Autodesk Fusion 360 part; units mm, degrees
note: some values were not read from the file. Chosen so that the rebuilt part matches the saved one: which bodies a step acts on.
(part 5 of 5)
sketch "スケッチ4 (17)" plane through (0, 0, 0) normal (0, 0, 1) x (1, 0, 0) in component "Stage2_Internal_Ring_Gear"
  circle A0 centre (62, 0) radius 3
  circle A1 centre (43.8406, 43.8406) radius 3
  circle A2 centre (0, 62) radius 3
  circle A3 centre (-43.8406, 43.8406) radius 3
  circle A4 centre (-62, 0) radius 3
  circle A5 centre (-43.8406, -43.8406) radius 3
  circle A6 centre (0, -62) radius 3
  circle A7 centre (43.8406, -43.8406) radius 3
extrude "Stage2_Ring_Bolt_Hole_Cut" cut sketch "スケッチ4 (17)" along normal blind 8 from surface at 76 bodies 19 in component "Stage2_Internal_Ring_Gear"
sketch "スケッチ5 (8)" plane through (0, 0, 0) normal (0, 0, 1) x (1, 0, 0) in component "Stage2_Internal_Ring_Gear"
  circle A0 centre (51.1941, 13.7174) radius 3.5
  circle A1 centre (37.4767, 37.4767) radius 3.5
  circle A2 centre (13.7174, 51.1941) radius 3.5
  circle A3 centre (-13.7174, 51.1941) radius 3.5
  circle A4 centre (-37.4767, 37.4767) radius 3.5
  circle A5 centre (-51.1941, 13.7174) radius 3.5
  circle A6 centre (-51.1941, -13.7174) radius 3.5
  circle A7 centre (-37.4767, -37.4767) radius 3.5
  circle A8 centre (-13.7174, -51.1941) radius 3.5
  circle A9 centre (13.7174, -51.1941) radius 3.5
  circle A10 centre (37.4767, -37.4767) radius 3.5
  circle A11 centre (51.1941, -13.7174) radius 3.5
extrude "Stage2_Ring_Lightening_Cut" cut sketch "スケッチ5 (8)" along normal blind 15 from surface at 73 bodies 19 in component "Stage2_Internal_Ring_Gear"
sketch "スケッチ1 (19)" plane through (0, 0, 0) normal (0, 0, 1) x (1, 0, 0) in component "Stage2_Output_Carrier"
  circle A0 centre (0, 0) radius 38
extrude "Stage2_Carrier_Lower_Plate_Extrude" add sketch "スケッチ1 (19)" along normal blind 5 from surface at 66 separate body makes body 20 in component "Stage2_Output_Carrier"
sketch "スケッチ2 (19)" plane through (0, 0, 0) normal (0, 0, 1) x (1, 0, 0) in component "Stage2_Output_Carrier"
  circle A0 centre (0, 0) radius 16
extrude "Stage2_Carrier_Lower_Bore_Cut" cut sketch "スケッチ2 (19)" along normal blind 7 from surface at 65 bodies 20 in component "Stage2_Output_Carrier"
sketch "スケッチ3 (18)" plane through (0, 0, 0) normal (0, 0, 1) x (1, 0, 0) in component "Stage2_Output_Carrier"
  circle A0 centre (21.2132, 21.2132) radius 5.5
  circle A1 centre (-21.2132, 21.2132) radius 5.5
  circle A2 centre (-21.2132, -21.2132) radius 5.5
  circle A3 centre (21.2132, -21.2132) radius 5.5
extrude "Stage2_Carrier_Post_Extrude" add sketch "スケッチ3 (18)" along normal blind 19 from surface at 71 bodies 20 in component "Stage2_Output_Carrier"
sketch "スケッチ4 (18)" plane through (0, 0, 0) normal (0, 0, 1) x (1, 0, 0) in component "Stage2_Output_Carrier"
  circle A0 centre (0, 0) radius 38
extrude "Stage2_Carrier_Output_Plate_Extrude" add sketch "スケッチ4 (18)" along normal blind 7 from surface at 90 bodies 20 in component "Stage2_Output_Carrier"
sketch "スケッチ5 (9)" plane through (0, 0, 0) normal (0, 0, 1) x (1, 0, 0) in component "Stage2_Output_Carrier"
  circle A0 centre (0, 0) radius 18
extrude "Stage2_Carrier_Hub_Extrude" add sketch "スケッチ5 (9)" along normal blind 6 from surface at 97 bodies 20 in component "Stage2_Output_Carrier"
sketch "スケッチ6 (4)" plane through (0, 0, 0) normal (0, 0, 1) x (1, 0, 0) in component "Stage2_Output_Carrier"
  circle A0 centre (35.1074, 14.542) radius 6
  circle A1 centre (14.542, 35.1074) radius 6
  circle A2 centre (-14.542, 35.1074) radius 6
  circle A3 centre (-35.1074, 14.542) radius 6
  circle A4 centre (-35.1074, -14.542) radius 6
  circle A5 centre (-14.542, -35.1074) radius 6
  circle A6 centre (14.542, -35.1074) radius 6
  circle A7 centre (35.1074, -14.542) radius 6
extrude "Stage2_Carrier_Lightening_Cut" cut sketch "スケッチ6 (4)" along normal blind 33 from surface at 65 bodies 20 in component "Stage2_Output_Carrier"
sketch "スケッチ7 (3)" plane through (0, 0, 0) normal (0, 0, 1) x (1, 0, 0) in component "Stage2_Output_Carrier"
  circle A0 centre (30, 0) radius 4.1
  circle A1 centre (0, 30) radius 4.1
  circle A2 centre (-30, 0) radius 4.1
  circle A3 centre (0, -30) radius 4.1
extrude "Stage2_Carrier_Pin_Hole_Cut" cut sketch "スケッチ7 (3)" along normal blind 33 from surface at 65 bodies 20 in component "Stage2_Output_Carrier"
sketch "スケッチ1 (20)" plane through (0, 0, 0) normal (0, 0, 1) x (1, 0, 0) in component "Output_Shaft"
  circle A0 centre (0, 0) radius 12
extrude "Output_Shaft_Main_Extrude" add sketch "スケッチ1 (20)" along normal blind 35 from surface at 99 separate body makes body 21 in component "Output_Shaft"
sketch "スケッチ2 (20)" plane through (0, 0, 0) normal (0, 0, 1) x (1, 0, 0) in component "Output_Shaft"
  circle A0 centre (0, 0) radius 15
extrude "Output_Shaft_Bearing_Seat_Extrude" add sketch "スケッチ2 (20)" along normal blind 10 from surface at 106 bodies 21 in component "Output_Shaft"
sketch "スケッチ3 (19)" plane through (0, 0, 0) normal (0, 0, 1) x (1, 0, 0) in component "Output_Shaft"
  line L0 (-3, 10) -> (3, 10)
  line L1 (3, 10) -> (3, 12.5)
  line L2 (3, 12.5) -> (-3, 12.5)
  line L3 (-3, 12.5) -> (-3, 10)
extrude "Output_Shaft_Keyway_Cut" cut sketch "スケッチ3 (19)" along normal blind 15 from surface at 119 bodies 21 in component "Output_Shaft"
sketch "スケッチ1 (21)" plane through (0, 0, 0) normal (0, 0, 1) x (1, 0, 0) in component "Output_Flange"
  circle A0 centre (0, 0) radius 18
extrude "Output_Flange_Hub_Extrude" add sketch "スケッチ1 (21)" along normal blind 6 from surface at 128 separate body makes body 22 in component "Output_Flange"
sketch "スケッチ2 (21)" plane through (0, 0, 0) normal (0, 0, 1) x (1, 0, 0) in component "Output_Flange"
  circle A0 centre (0, 0) radius 40
extrude "Output_Flange_Plate_Extrude" add sketch "スケッチ2 (21)" along normal blind 8 from surface at 134 bodies 22 in component "Output_Flange"
sketch "スケッチ3 (20)" plane through (0, 0, 0) normal (0, 0, 1) x (1, 0, 0) in component "Output_Flange"
  circle A0 centre (0, 0) radius 12.15
extrude "Output_Flange_Bore_Cut" cut sketch "スケッチ3 (20)" along normal blind 10 from surface at 127 bodies 22 in component "Output_Flange"
sketch "スケッチ4 (19)" plane through (0, 0, 0) normal (0, 0, 1) x (1, 0, 0) in component "Output_Flange"
  circle A0 centre (32, 0) radius 4
  circle A1 centre (22.6274, 22.6274) radius 4
  circle A2 centre (0, 32) radius 4
  circle A3 centre (-22.6274, 22.6274) radius 4
  circle A4 centre (-32, 0) radius 4
  circle A5 centre (-22.6274, -22.6274) radius 4
  circle A6 centre (0, -32) radius 4
  circle A7 centre (22.6274, -22.6274) radius 4
extrude "Output_Flange_Bolt_Hole_Cut" cut sketch "スケッチ4 (19)" along normal blind 10 from surface at 133 bodies 22 in component "Output_Flange"
sketch "スケッチ5 (10)" plane through (0, 0, 0) normal (0, 0, 1) x (1, 0, 0) in component "Output_Flange"
  circle A0 centre (21.2504, 5.694) radius 2.5
  circle A1 centre (15.5563, 15.5563) radius 2.5
  circle A2 centre (5.694, 21.2504) radius 2.5
  circle A3 centre (-5.694, 21.2504) radius 2.5
  circle A4 centre (-15.5563, 15.5563) radius 2.5
  circle A5 centre (-21.2504, 5.694) radius 2.5
  circle A6 centre (-21.2504, -5.694) radius 2.5
  circle A7 centre (-15.5563, -15.5563) radius 2.5
  circle A8 centre (-5.694, -21.2504) radius 2.5
  circle A9 centre (5.694, -21.2504) radius 2.5
  circle A10 centre (15.5563, -15.5563) radius 2.5
  circle A11 centre (21.2504, -5.694) radius 2.5
extrude "Output_Flange_Index_Hole_Cut" cut sketch "スケッチ5 (10)" along normal blind 10 from surface at 133 bodies 22 in component "Output_Flange"
sketch "スケッチ8" plane through (0, 0, 0) normal (0, 0, 1) x (1, 0, 0) in component "Lower_Base_Plate"
  circle A0 centre (0, 0) radius 22.3
extrude "Base_Bearing_Counterbore_Cut" cut sketch "スケッチ8" along normal blind 7 from surface at 13 bodies 1 in component "Lower_Base_Plate"
sketch "スケッチ8 (2)" plane through (0, 0, 0) normal (0, 0, 1) x (1, 0, 0) in component "Stage1_Planet_Carrier"
  circle A0 centre (0, 0) radius 23
extrude "Stage1_Carrier_Bore_Relief_Cut" cut sketch "スケッチ8 (2)" along normal blind 8 from surface at 23 bodies 11 in component "Stage1_Planet_Carrier"
sketch "スケッチ1 (22)" plane through (0, 0, 0) normal (0, 0, 1) x (1, 0, 0) in component "Bearing_Set"
  circle A0 centre (0, 0) radius 22
extrude "Input_Bearing_Outer_Race_Extrude" add sketch "スケッチ1 (22)" along normal blind 10 from surface at 15 separate body makes body 23 in component "Bearing_Set"
sketch "スケッチ2 (22)" plane through (0, 0, 0) normal (0, 0, 1) x (1, 0, 0) in component "Bearing_Set"
  circle A0 centre (0, 0) radius 20.6
extrude "Input_Bearing_Outer_Race_Bore_Cut" cut sketch "スケッチ2 (22)" along normal blind 12 from surface at 14 bodies 23 in component "Bearing_Set"
sketch "スケッチ3 (21)" plane through (0, 0, 0) normal (0, 0, 1) x (1, 0, 0) in component "Bearing_Set"
  circle A0 centre (0, 0) radius 20.4
extrude "Input_Bearing_Cage_Extrude" add sketch "スケッチ3 (21)" along normal blind 6 from surface at 17 separate body makes body 24 in component "Bearing_Set"
sketch "スケッチ4 (20)" plane through (0, 0, 0) normal (0, 0, 1) x (1, 0, 0) in component "Bearing_Set"
  circle A0 centre (0, 0) radius 18.6
extrude "Input_Bearing_Cage_Bore_Cut" cut sketch "スケッチ4 (20)" along normal blind 8 from surface at 16 bodies 24 in component "Bearing_Set"
sketch "スケッチ5 (11)" plane through (0, 0, 0) normal (0, 0, 1) x (1, 0, 0) in component "Bearing_Set"
  circle A0 centre (0, 0) radius 18.4
extrude "Input_Bearing_Inner_Race_Extrude" add sketch "スケッチ5 (11)" along normal blind 10 from surface at 15 separate body makes body 25 in component "Bearing_Set"
sketch "スケッチ6 (5)" plane through (0, 0, 0) normal (0, 0, 1) x (1, 0, 0) in component "Bearing_Set"
  circle A0 centre (0, 0) radius 13.1
extrude "Input_Bearing_Inner_Race_Bore_Cut" cut sketch "スケッチ6 (5)" along normal blind 12 from surface at 14 bodies 25 in component "Bearing_Set"
sketch "スケッチ7 (4)" plane through (0, 0, 0) normal (0, 0, 1) x (1, 0, 0) in component "Bearing_Set"
  circle A0 centre (0, 0) radius 23.8
extrude "Intermediate_Bearing_Outer_Race_Extrude" add sketch "スケッチ7 (4)" along normal blind 6 from surface at 57 separate body makes body 26 in component "Bearing_Set"
sketch "スケッチ8 (3)" plane through (0, 0, 0) normal (0, 0, 1) x (1, 0, 0) in component "Bearing_Set"
  circle A0 centre (0, 0) radius 22.4
extrude "Intermediate_Bearing_Outer_Race_Bore_Cut" cut sketch "スケッチ8 (3)" along normal blind 8 from surface at 56 bodies 26 in component "Bearing_Set"
sketch "スケッチ9" plane through (0, 0, 0) normal (0, 0, 1) x (1, 0, 0) in component "Bearing_Set"
  circle A0 centre (0, 0) radius 22.2
extrude "Intermediate_Bearing_Cage_Extrude" add sketch "スケッチ9" along normal blind 4 from surface at 58 separate body makes body 27 in component "Bearing_Set"
sketch "スケッチ10" plane through (0, 0, 0) normal (0, 0, 1) x (1, 0, 0) in component "Bearing_Set"
  circle A0 centre (0, 0) radius 20.4
extrude "Intermediate_Bearing_Cage_Bore_Cut" cut sketch "スケッチ10" along normal blind 6 from surface at 57 bodies 27 in component "Bearing_Set"
sketch "スケッチ11" plane through (0, 0, 0) normal (0, 0, 1) x (1, 0, 0) in component "Bearing_Set"
  circle A0 centre (0, 0) radius 20.2
extrude "Intermediate_Bearing_Inner_Race_Extrude" add sketch "スケッチ11" along normal blind 6 from surface at 57 separate body makes body 28 in component "Bearing_Set"
sketch "スケッチ12" plane through (0, 0, 0) normal (0, 0, 1) x (1, 0, 0) in component "Bearing_Set"
  circle A0 centre (0, 0) radius 16.2
extrude "Intermediate_Bearing_Inner_Race_Bore_Cut" cut sketch "スケッチ12" along normal blind 8 from surface at 56 bodies 28 in component "Bearing_Set"
sketch "スケッチ13" plane through (0, 0, 0) normal (0, 0, 1) x (1, 0, 0) in component "Bearing_Set"
  circle A0 centre (0, 0) radius 23.5
extrude "Output_Bearing_Outer_Race_Extrude" add sketch "スケッチ13" along normal blind 10 from surface at 106 separate body makes body 29 in component "Bearing_Set"
sketch "スケッチ14" plane through (0, 0, 0) normal (0, 0, 1) x (1, 0, 0) in component "Bearing_Set"
  circle A0 centre (0, 0) radius 22.1
extrude "Output_Bearing_Outer_Race_Bore_Cut" cut sketch "スケッチ14" along normal blind 12 from surface at 105 bodies 29 in component "Bearing_Set"
sketch "スケッチ15" plane through (0, 0, 0) normal (0, 0, 1) x (1, 0, 0) in component "Bearing_Set"
  circle A0 centre (0, 0) radius 21.9
extrude "Output_Bearing_Cage_Extrude" add sketch "スケッチ15" along normal blind 6 from surface at 108 separate body makes body 30 in component "Bearing_Set"
sketch "スケッチ16" plane through (0, 0, 0) normal (0, 0, 1) x (1, 0, 0) in component "Bearing_Set"
  circle A0 centre (0, 0) radius 20.1
extrude "Output_Bearing_Cage_Bore_Cut" cut sketch "スケッチ16" along normal blind 8 from surface at 107 bodies 30 in component "Bearing_Set"
sketch "スケッチ17" plane through (0, 0, 0) normal (0, 0, 1) x (1, 0, 0) in component "Bearing_Set"
  circle A0 centre (0, 0) radius 19.9
extrude "Output_Bearing_Inner_Race_Extrude" add sketch "スケッチ17" along normal blind 10 from surface at 106 separate body makes body 31 in component "Bearing_Set"
sketch "スケッチ18" plane through (0, 0, 0) normal (0, 0, 1) x (1, 0, 0) in component "Bearing_Set"
  circle A0 centre (0, 0) radius 15.1
extrude "Output_Bearing_Inner_Race_Bore_Cut" cut sketch "スケッチ18" along normal blind 12 from surface at 105 bodies 31 in component "Bearing_Set"
sketch "スケッチ1 (23)" plane through (0, 0, 0) normal (0, 0, 1) x (1, 0, 0) in component "Planet_Pin_Set"
  circle A0 centre (31.5, 0) radius 4
  circle A1 centre (-15.75, 27.2798) radius 4
  circle A2 centre (-15.75, -27.2798) radius 4
extrude "Stage1_Planet_Pin_Extrude" add sketch "スケッチ1 (23)" along normal blind 35.8 from surface at 22 separate body makes body 32 at (35.4801, -0.3983, 33.9333) makes body 33 at (-11.7699, 26.8815, 33.9333) makes body 34 at (-11.7699, -27.6781, 33.9333) in component "Planet_Pin_Set"
sketch "スケッチ2 (23)" plane through (0, 0, 0) normal (0, 0, 1) x (1, 0, 0) in component "Planet_Pin_Set"
  circle A0 centre (31.5, 0) radius 8
  circle A1 centre (-15.75, 27.2798) radius 8
  circle A2 centre (-15.75, -27.2798) radius 8
extrude "Stage1_Pin_Washer_Lower_Extrude" add sketch "スケッチ2 (23)" along normal blind 2 from surface at 20 bodies 32 33 34 in component "Planet_Pin_Set"
sketch "スケッチ3 (22)" plane through (0, 0, 0) normal (0, 0, 1) x (1, 0, 0) in component "Planet_Pin_Set"
  circle A0 centre (31.5, 0) radius 6.5
  circle A1 centre (-15.75, 27.2798) radius 6.5
  circle A2 centre (-15.75, -27.2798) radius 6.5
extrude "Stage1_Pin_Collar_Upper_Extrude" add sketch "スケッチ3 (22)" along normal blind 1.8 from surface at 56 bodies 32 33 34 in component "Planet_Pin_Set"
sketch "スケッチ4 (21)" plane through (0, 0, 0) normal (0, 0, 1) x (1, 0, 0) in component "Planet_Pin_Set"
  circle A0 centre (30, 0) radius 4
  circle A1 centre (0, 30) radius 4
  circle A2 centre (-30, 0) radius 4
  circle A3 centre (0, -30) radius 4
extrude "Stage2_Planet_Pin_Extrude" add sketch "スケッチ4 (21)" along normal blind 33 from surface at 64 separate body makes body 35 at (-26.0199, -0.3983, 86) makes body 36 at (3.9801, 29.6017, 86) makes body 37 at (33.9801, -0.3983, 86) makes body 38 at (3.9801, -30.3983, 86) in component "Planet_Pin_Set"
sketch "スケッチ5 (12)" plane through (0, 0, 0) normal (0, 0, 1) x (1, 0, 0) in component "Planet_Pin_Set"
  circle A0 centre (30, 0) radius 8
  circle A1 centre (0, 30) radius 8
  circle A2 centre (-30, 0) radius 8
  circle A3 centre (0, -30) radius 8
extrude "Stage2_Pin_Washer_Lower_Extrude" add sketch "スケッチ5 (12)" along normal blind 2 from surface at 62 bodies 32 33 34 35 36 37 38 in component "Planet_Pin_Set"
sketch "スケッチ6 (6)" plane through (0, 0, 0) normal (0, 0, 1) x (1, 0, 0) in component "Planet_Pin_Set"
  line L0 (36.6, 0) -> (33.3, 5.7158)
  line L1 (33.3, 5.7158) -> (26.7, 5.7158)
  line L2 (26.7, 5.7158) -> (23.4, 0)
  line L3 (23.4, 0) -> (26.7, -5.7158)
  line L4 (26.7, -5.7158) -> (33.3, -5.7158)
  line L5 (33.3, -5.7158) -> (36.6, 0)
  line L6 (6.6, 30) -> (3.3, 35.7158)
  line L7 (3.3, 35.7158) -> (-3.3, 35.7158)
  line L8 (-3.3, 35.7158) -> (-6.6, 30)
  line L9 (-6.6, 30) -> (-3.3, 24.2842)
  line L10 (-3.3, 24.2842) -> (3.3, 24.2842)
  line L11 (3.3, 24.2842) -> (6.6, 30)
  line L12 (-23.4, 0) -> (-26.7, 5.7158)
  line L13 (-26.7, 5.7158) -> (-33.3, 5.7158)
  line L14 (-33.3, 5.7158) -> (-36.6, 0)
  line L15 (-36.6, 0) -> (-33.3, -5.7158)
  line L16 (-33.3, -5.7158) -> (-26.7, -5.7158)
  line L17 (-26.7, -5.7158) -> (-23.4, 0)
  line L18 (6.6, -30) -> (3.3, -24.2842)
  line L19 (3.3, -24.2842) -> (-3.3, -24.2842)
  line L20 (-3.3, -24.2842) -> (-6.6, -30)
  line L21 (-6.6, -30) -> (-3.3, -35.7158)
  line L22 (-3.3, -35.7158) -> (3.3, -35.7158)
  line L23 (3.3, -35.7158) -> (6.6, -30)
extrude "Stage2_Pin_Nut_Extrude" add sketch "スケッチ6 (6)" along normal blind 5 from surface at 97 bodies 32 33 34 35 36 37 38 in component "Planet_Pin_Set"
sketch "スケッチ1 (24)" plane through (0, 0, 0) normal (0, 0, 1) x (1, 0, 0) in component "Housing_Tie_Rods"
  circle A0 centre (75, 0) radius 4
extrude "Housing_TieRod_Extrude" add sketch "スケッチ1 (24)" along normal blind 101 from surface at 14 separate body makes body 39 in component "Housing_Tie_Rods"
pattern_circular "Housing_TieRod_Pattern" count 8 over 360 about axis through (0, 0, 1.75) along (0, 0, 1) of bodies 39 makes body 40 at (55.9989, 55.7169, 81.3333) makes body 41 at (0.1994, 78.995, 81.3333) makes body 42 at (-55.7169, 55.9989, 81.3333) makes body 43 at (-78.995, 0.1994, 81.3333) makes body 44 at (-55.9989, -55.7169, 81.3333) makes body 45 at (-0.1994, -78.995, 81.3333) makes body 46 at (55.7169, -55.9989, 81.3333) in component "Housing_Tie_Rods"
sketch "スケッチ1 (25)" plane through (0, 0, 0) normal (0, 0, 1) x (1, 0, 0) in component "Fastener_Set"
  circle A0 centre (75, 0) radius 9
extrude "TieRod_Lower_Washer_Extrude" add sketch "スケッチ1 (25)" along normal blind 1.6 from surface at 20 separate body makes body 47 in component "Fastener_Set"
sketch "スケッチ2 (24)" plane through (0, 0, 0) normal (0, 0, 1) x (1, 0, 0) in component "Fastener_Set"
  line L0 (83.1, 0) -> (79.05, 7.0148)
  line L1 (79.05, 7.0148) -> (70.95, 7.0148)
  line L2 (70.95, 7.0148) -> (66.9, 0)
  line L3 (66.9, 0) -> (70.95, -7.0148)
  line L4 (70.95, -7.0148) -> (79.05, -7.0148)
  line L5 (79.05, -7.0148) -> (83.1, 0)
extrude "TieRod_Lower_Nut_Extrude" add sketch "スケッチ2 (24)" along normal blind 7 from surface at 21.6 separate body makes body 48 in component "Fastener_Set"
sketch "スケッチ3 (23)" plane through (0, 0, 0) normal (0, 0, 1) x (1, 0, 0) in component "Fastener_Set"
  circle A0 centre (75, 0) radius 9
extrude "TieRod_Upper_Washer_Extrude" add sketch "スケッチ3 (23)" along normal blind 1.6 from surface at 104 separate body makes body 49 in component "Fastener_Set"
sketch "スケッチ4 (22)" plane through (0, 0, 0) normal (0, 0, 1) x (1, 0, 0) in component "Fastener_Set"
  line L0 (83.1, 0) -> (79.05, 7.0148)
  line L1 (79.05, 7.0148) -> (70.95, 7.0148)
  line L2 (70.95, 7.0148) -> (66.9, 0)
  line L3 (66.9, 0) -> (70.95, -7.0148)
  line L4 (70.95, -7.0148) -> (79.05, -7.0148)
  line L5 (79.05, -7.0148) -> (83.1, 0)
extrude "TieRod_Upper_Nut_Extrude" add sketch "スケッチ4 (22)" along normal blind 7 from surface at 105.6 separate body makes body 50 in component "Fastener_Set"
pattern_circular "Fastener_Circular_Pattern" count 8 over 360 about axis through (0, 0, 1.75) along (0, 0, 1) of bodies 47 48 49 50 makes body 51 at (48.1121, 50.7772, 20) makes body 52 at (2.4777, 78.6341, 20) makes body 53 at (-51.2227, 48.0619, 20) makes body 54 at (-78.6341, 2.4777, 20) makes body 55 at (-49.9226, -53.9664, 20) makes body 56 at (-2.4777, -78.6341, 20) makes body 57 at (50.7772, -48.1121, 20) makes body 58 at (52.3342, 55.641, 28.6) makes body 59 at (-2.3383, 76.35, 28.6) makes body 60 at (-53.7318, 50.425, 28.6) makes body 61 at (-76.35, -2.3383, 28.6) makes body 62 at (-52.3342, -55.641, 28.6) makes body 63 at (2.3383, -76.35, 28.6) makes body 64 at (55.641, -52.3342, 28.6) makes body 65 at (48.1121, 50.7772, 104) makes body 66 at (2.4777, 78.6341, 104) makes body 67 at (-51.2227, 48.0619, 104) makes body 68 at (-78.6341, 2.4777, 104) makes body 69 at (-49.9226, -53.9664, 104) makes body 70 at (-2.4777, -78.6341, 104) makes body 71 at (50.7772, -48.1121, 104) makes body 72 at (52.3342, 55.641, 112.6) makes body 73 at (-2.3383, 76.35, 112.6) makes body 74 at (-53.7318, 50.425, 112.6) makes body 75 at (-76.35, -2.3383, 112.6) makes body 76 at (-52.3342, -55.641, 112.6) makes body 77 at (2.3383, -76.35, 112.6) makes body 78 at (55.641, -52.3342, 112.6) in component "Fastener_Set"
sketch "スケッチ1 (26)" plane through (0, 0, 0) normal (0, 0, 1) x (1, 0, 0) in component "Transparent_Outer_Housing"
  circle A0 centre (0, 0) radius 69
extrude "Outer_Housing_Wall_Extrude" add sketch "スケッチ1 (26)" along normal blind 74 from surface at 30 separate body makes body 79 in component "Transparent_Outer_Housing"
sketch "スケッチ2 (25)" plane through (0, 0, 0) normal (0, 0, 1) x (1, 0, 0) in component "Transparent_Outer_Housing"
  circle A0 centre (0, 0) radius 80
extrude "Outer_Housing_Lower_Flange_Extrude" add sketch "スケッチ2 (25)" along normal blind 8 from surface at 30 bodies 79 in component "Transparent_Outer_Housing"
sketch "スケッチ3 (24)" plane through (0, 0, 0) normal (0, 0, 1) x (1, 0, 0) in component "Transparent_Outer_Housing"
  circle A0 centre (0, 0) radius 80
extrude "Outer_Housing_Upper_Flange_Extrude" add sketch "スケッチ3 (24)" along normal blind 8 from surface at 96 bodies 79 in component "Transparent_Outer_Housing"
sketch "スケッチ4 (23)" plane through (0, 0, 0) normal (0, 0, 1) x (1, 0, 0) in component "Transparent_Outer_Housing"
  line L0 (62.3154, 22.0235) -> (68.7826, 24.7023)
  line L1 (68.7826, 24.7023) -> (66.1038, 31.1695)
  line L2 (66.1038, 31.1695) -> (59.6367, 28.4907)
  line L3 (59.6367, 28.4907) -> (62.3154, 22.0235)
  line L4 (28.4907, 59.6367) -> (31.1695, 66.1038)
  line L5 (31.1695, 66.1038) -> (24.7023, 68.7826)
  line L6 (24.7023, 68.7826) -> (22.0235, 62.3154)
  line L7 (22.0235, 62.3154) -> (28.4907, 59.6367)
  line L8 (-22.0235, 62.3154) -> (-24.7023, 68.7826)
  line L9 (-24.7023, 68.7826) -> (-31.1695, 66.1038)
  line L10 (-31.1695, 66.1038) -> (-28.4907, 59.6367)
  line L11 (-28.4907, 59.6367) -> (-22.0235, 62.3154)
  line L12 (-59.6367, 28.4907) -> (-66.1038, 31.1695)
  line L13 (-66.1038, 31.1695) -> (-68.7826, 24.7023)
  line L14 (-68.7826, 24.7023) -> (-62.3154, 22.0235)
  line L15 (-62.3154, 22.0235) -> (-59.6367, 28.4907)
  line L16 (-62.3154, -22.0235) -> (-68.7826, -24.7023)
  line L17 (-68.7826, -24.7023) -> (-66.1038, -31.1695)
  line L18 (-66.1038, -31.1695) -> (-59.6367, -28.4907)
  line L19 (-59.6367, -28.4907) -> (-62.3154, -22.0235)
  line L20 (-28.4907, -59.6367) -> (-31.1695, -66.1038)
  line L21 (-31.1695, -66.1038) -> (-24.7023, -68.7826)
  line L22 (-24.7023, -68.7826) -> (-22.0235, -62.3154)
  line L23 (-22.0235, -62.3154) -> (-28.4907, -59.6367)
  line L24 (22.0235, -62.3154) -> (24.7023, -68.7826)
  line L25 (24.7023, -68.7826) -> (31.1695, -66.1038)
  line L26 (31.1695, -66.1038) -> (28.4907, -59.6367)
  line L27 (28.4907, -59.6367) -> (22.0235, -62.3154)
  line L28 (59.6367, -28.4907) -> (66.1038, -31.1695)
  line L29 (66.1038, -31.1695) -> (68.7826, -24.7023)
  line L30 (68.7826, -24.7023) -> (62.3154, -22.0235)
  line L31 (62.3154, -22.0235) -> (59.6367, -28.4907)
extrude "Outer_Housing_Rib_Extrude" add sketch "スケッチ4 (23)" along normal blind 58 from surface at 38 bodies 79 in component "Transparent_Outer_Housing"
sketch "スケッチ5 (13)" plane through (0, 0, 0) normal (0, 0, 1) x (1, 0, 0) in component "Transparent_Outer_Housing"
  circle A0 centre (0, 0) radius 66
extrude "Outer_Housing_Bore_Cut" cut sketch "スケッチ5 (13)" along normal blind 76 from surface at 29 bodies 79 in component "Transparent_Outer_Housing"
sketch "スケッチ6 (7)" plane through (0, 0, 0) normal (0, 0, 1) x (1, 0, 0) in component "Transparent_Outer_Housing"
  circle A0 centre (75, 0) radius 4.6
  circle A1 centre (53.033, 53.033) radius 4.6
  circle A2 centre (0, 75) radius 4.6
  circle A3 centre (-53.033, 53.033) radius 4.6
  circle A4 centre (-75, 0) radius 4.6
  circle A5 centre (-53.033, -53.033) radius 4.6
  circle A6 centre (0, -75) radius 4.6
  circle A7 centre (53.033, -53.033) radius 4.6
extrude "Outer_Housing_Bolt_Hole_Cut" cut sketch "スケッチ6 (7)" along normal blind 76 from surface at 29 bodies 79 in component "Transparent_Outer_Housing"
fillet "Base_Plate_Edge_Fillet" radius 3 2 edges at (-78.3155, -30.3757, 14) (-78.3155, -30.3757, 0) on bodies 1 in component "Lower_Base_Plate"
fillet "Output_Flange_Edge_Fillet" radius 2 2 edges at (-37.2931, -14.4646, 134) (-37.2931, -14.4646, 142) on bodies 22 in component "Output_Flange"
component "Lower_Base_Plate" placed x (1, 0, 0) y (0, 1, 0) z (0, 0, 1) at (0, 0, 0)
component "Lower_Housing_Ring" placed x (1, 0, 0) y (0, 1, 0) z (0, 0, 1) at (0, 0, 0)
component "Stage1_Sun_Gear" placed x (1, 0, 0) y (0, 1, 0) z (0, 0, 1) at (0, 0, 0)
component "Stage1_Planet_Gear_A" placed x (1, 0, 0) y (0, 1, 0) z (0, 0, 1) at (0, 0, 0)
component "Stage1_Planet_Gear_B" placed x (1, 0, 0) y (0, 1, 0) z (0, 0, 1) at (0, 0, 0)
component "Stage1_Planet_Gear_C" placed x (1, 0, 0) y (0, 1, 0) z (0, 0, 1) at (0, 0, 0)
component "Stage1_Internal_Ring_Gear" placed x (1, 0, 0) y (0, 1, 0) z (0, 0, 1) at (0, 0, 0)
component "Input_Shaft" placed x (1, 0, 0) y (0, 1, 0) z (0, 0, 1) at (0, 0, 0)
component "Input_Handwheel" placed x (1, 0, 0) y (0, 1, 0) z (0, 0, 1) at (0, 0, 0)
component "Stage1_Planet_Carrier" placed x (1, 0, 0) y (0, 1, 0) z (0, 0, 1) at (0, 0, 0)
component "Intermediate_Shaft" placed x (1, 0, 0) y (0, 1, 0) z (0, 0, 1) at (0, 0, 0)
component "Stage_Separator_Plate" placed x (1, 0, 0) y (0, 1, 0) z (0, 0, 1) at (0, 0, 0)
component "Stage2_Sun_Gear" placed x (1, 0, 0) y (0, 1, 0) z (0, 0, 1) at (0, 0, 0)
component "Stage2_Planet_Gear_A" placed x (1, 0, 0) y (0, 1, 0) z (0, 0, 1) at (0, 0, 0)
component "Stage2_Planet_Gear_B" placed x (1, 0, 0) y (0, 1, 0) z (0, 0, 1) at (0, 0, 0)
component "Stage2_Planet_Gear_C" placed x (1, 0, 0) y (0, 1, 0) z (0, 0, 1) at (0, 0, 0)
component "Stage2_Planet_Gear_D" placed x (1, 0, 0) y (0, 1, 0) z (0, 0, 1) at (0, 0, 0)
component "Stage2_Internal_Ring_Gear" placed x (1, 0, 0) y (0, 1, 0) z (0, 0, 1) at (0, 0, 0)
component "Stage2_Output_Carrier" placed x (1, 0, 0) y (0, 1, 0) z (0, 0, 1) at (0, 0, 0)
component "Output_Shaft" placed x (1, 0, 0) y (0, 1, 0) z (0, 0, 1) at (0, 0, 0)
component "Output_Flange" placed x (1, 0, 0) y (0, 1, 0) z (0, 0, 1) at (0, 0, 0)
component "Bearing_Set" placed x (1, 0, 0) y (0, 1, 0) z (0, 0, 1) at (0, 0, 0)
component "Planet_Pin_Set" placed x (1, 0, 0) y (0, 1, 0) z (0, 0, 1) at (0, 0, 0)
component "Housing_Tie_Rods" placed x (1, 0, 0) y (0, 1, 0) z (0, 0, 1) at (0, 0, 0)
component "Fastener_Set" placed x (1, 0, 0) y (0, 1, 0) z (0, 0, 1) at (0, 0, 0)
component "Transparent_Outer_Housing" placed x (1, 0, 0) y (0, 1, 0) z (0, 0, 1) at (0, 0, 0)
equation "GearModule = 1.5 mm"
equation "GearFaceWidth = 12.0 mm"
equation "BasePlateThickness = 14.0 mm"
equation "Stage1_GearPlane = 34.0 mm"
equation "Stage2_GearPlane = 74 mm"
equation "HousingInnerRadius = 66.0 mm"
equation "StageSpacing = 40 mm"
equation "TieRodRadius = 75.0 mm"
equation "d10 = BasePlateThickness"
equation "d45 = Stage1_GearPlane"
equation "d46 = GearFaceWidth"
equation "d60 = Stage1_GearPlane"
equation "d61 = GearFaceWidth"
equation "d72 = Stage1_GearPlane"
equation "d73 = GearFaceWidth"
equation "d84 = Stage1_GearPlane"
equation "d85 = GearFaceWidth"
equation "d183 = Stage2_GearPlane"
equation "d184 = GearFaceWidth"
equation "d195 = Stage2_GearPlane"
equation "d196 = GearFaceWidth"
equation "d207 = Stage2_GearPlane"
equation "d208 = GearFaceWidth"
equation "d219 = Stage2_GearPlane"
equation "d220 = GearFaceWidth"
equation "d231 = Stage2_GearPlane"
equation "d232 = GearFaceWidth"
equation "d243 = Stage2_GearPlane"
equation "d244 = GearFaceWidth"
named bodies: "Input_Bearing_Outer_Race", "Input_Bearing_Cage", "Input_Bearing_Inner_Race", "Intermediate_Bearing_Outer_Race", "Intermediate_Bearing_Cage", "Intermediate_Bearing_Inner_Race", "Output_Bearing_Outer_Race", "Output_Bearing_Cage", "Output_Bearing_Inner_Race"
